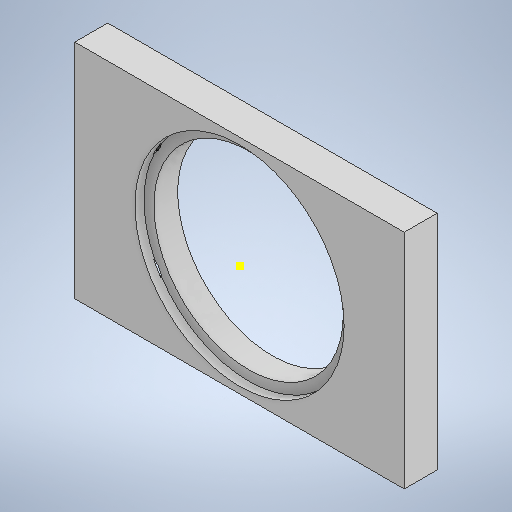
# Autodesk Inventor part: zhunzhiguan2
Saved by Autodesk Inventor 2025 (Build 290162000, 162)
## iProperties
Created: 2024-08-27
Part Number: zhunzhiguan2
Material: 常规
Document SubType Name: Sheet Metal
Designer: Leexi
Density: 1 g/cm^3
Sheet Metal Rule: 默认_mm
Appearance: 默认
Author: Leexi
Autodesk Inventor part; units mm, degrees
ref_plane "YZ Plane" through (0, 0, 0) normal (1, 0, 0) x (0, 1, 0)
ref_plane "XZ Plane" through (0, 0, 0) normal (0, 1, 0) x (-1, 0, 0)
ref_plane "XY Plane" through (0, 0, 0) normal (0, 0, 1) x (1, 0, 0)
sketch "草图1" plane through (0, 0, 0) normal (0, 0, 1) x (1, 0, 0)
  line L0 (-25.95, -15) -> (25.95, -15) construction
  line L1 (25.95, -15) -> (25.95, 15) construction
  line L2 (25.95, 15) -> (-25.95, 15) construction
  line L3 (-25.95, 15) -> (-25.95, -15) construction
  line L4 (-25.95, -15) -> (25.95, 15) construction
  line L5 (25.95, -15) -> (-25.95, 15) construction
  line L6 (0, 0) -> (-12.9865, 7.5067) construction
  line L7 (0, 0) -> (12.9865, 7.5067) construction
  line L8 (0, 0) -> (-12.9865, -7.5067) construction
  line L9 (0, 0) -> (12.9865, -7.5067) construction
  circle A0 centre (0, 0) radius 11.5
  line L10 (-20, -13.5) -> (20, -13.5)
  line L11 (20, -13.5) -> (20, 13.5)
  line L12 (20, 13.5) -> (-20, 13.5)
  line L13 (-20, 13.5) -> (-20, -13.5)
  line L14 (-20, -13.5) -> (20, 13.5) construction
  line L15 (20, -13.5) -> (-20, 13.5) construction
  circle A1 centre (12.9865, 7.5067) radius 2.5
  circle A2 centre (-12.9865, 7.5067) radius 2.5
  circle A3 centre (12.9865, -7.5067) radius 2.5
  dimension "d0" = 51.9
  dimension "d1" = 30
  dimension "d6" = 23
  dimension "d7" = 40
  dimension "d8" = 27
  dimension "d11" = 5
  dimension "d12" = 5
  dimension "d13" = 5
  constraints: 32 end point, 9 coincident, 4 centre point, 4 midpoint, 4 parallel, 4 point on line, 2 horizontal, 2 perpendicular
  measures "d0" distance of L0.start L0.end
  measures "d1" distance of L1.end L0.end
  measures "d6" diameter of A0
  measures "d7" distance of L10.start L10.end
  measures "d8" distance of L11.end L10.end
  measures "d11" diameter of A1
  measures "d12" diameter of A2
  measures "d13" diameter of A3
extrude "拉伸1" add sketch "草图1" along normal blind 4 contours L13 L12 L11 L10 | A1 | A2 | A3
hole "孔1" at (-12.9865, 7.5067, 0) at (12.9865, 7.5067, 0) at (12.9865, -7.5067, 0) at (-12.9865, -7.5067, 0) at (0, 0, 0) direction (0, 0, 1) diameter 4.94 depth 3
sketch "草图2" plane through (0, 0, 4) normal (0, 0, 1) x (1, 0, 0)
  point P0 (0, 0)
  point P1 (0, 0)
  constraints: 1 coincident
hole "孔2" at (0, 0, 4) direction (0, 0, -1) diameter 25.4 depth 1.1
sketch "草图3" plane through (0, 0, 4) normal (0, 0, 1) x (1, 0, 0)
  point P0 (0, 0)
equation "\"折弯半径\" = 厚度"
equation "\"折弯释压宽度\" = 厚度"
equation "\"折弯释压深度\" = 0.5 * 厚度"
equation "\"拐角释压尺寸\" = 4 * 厚度"
equation "\"最小余量\" = 2 * 厚度"
equation "\"过渡半径\" = 折弯半径"
equation "\"Jacobi半径尺寸\" = 折弯半径"
equation "\"间隙大小\" = 厚度"
equation "\"厚度\" = 0.5"
